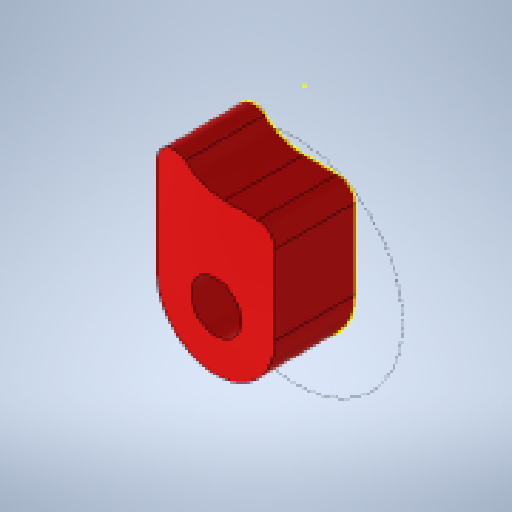
# Autodesk Inventor part: Cam - Lever
Saved by Autodesk Inventor 2023.2 (Build 272271000, 271)
## iProperties
Created: 2024-01-19
Part Number: Cam - Lever
Material: Nylon 6/6
Document SubType Name: Modeling
Designer: Nathan Cai
Density: 1.13 g/cm^3
Appearance: Red
Mass: 0.32887 g
Surface Area: 3.14473 cm^2
Volume: 0.291035 cm^3
Author: Nathan Cai
Autodesk Inventor part; units mm, degrees
ref_plane "YZ Plane" through (0, 0, 0) normal (1, 0, 0) x (0, 1, 0)
ref_plane "XZ Plane" through (0, 0, 0) normal (0, 1, 0) x (-1, 0, 0)
ref_plane "XY Plane" through (0, 0, 0) normal (0, 0, 1) x (1, 0, 0)
sketch "Sketch1" plane through (0, 0, 0) normal (0, 0, 1) x (1, 0, 0)
  circle A0 centre (0, 0) radius 1.5
  circle A1 centre (0, 0) radius 3.5
  circle A2 centre (0, 0) radius 5.75 construction
  line L0 (0, 0) -> (0, 5.75) construction
  circle A3 centre (0.5, 9.2365) radius 3.5
  line L1 (0, 0) -> (0, 5.75) construction
  line L2 (3.5, 0) -> (3.5, 5.75)
  line L3 (-3.5, 5.75) -> (-3.5, 0)
  arc A4 (-3.5, 0) -> (3.5, 0) centre (0, 0) ccw
  arc A5 (3.5, 5.75) -> (-1.9961, 2.875) centre (0, 5.75) ccw
  arc A6 (-3.4062, 0.805) -> (-3.4062, 4.945) centre (-12.1649, 2.875) ccw
  line L4 (0.5, 5.7365) -> (3.5, 5.7365)
  point P0 (0, 2.875)
  point P1 (-3.4345, 6.424)
  point P2 (3.5, 0)
  point P3 (3.244, 7.0639)
  point P4 (-3.5, 0)
  point P5 (-2.744, 7.9226)
  dimension "d2" = 11.5
  dimension "d3" = 7
  dimension "d0" = 3
  dimension "d1" = 7
  dimension "d4" = 3.5
  dimension "d9" = 0.5
  dimension "d10" = 9
  constraints: 12 end point, 11 point on circle, 6 tangent, 5 centre point, 3 coincident, 2 equal length, 1 horizontal, 1 midpoint, 1 perpendicular, 1 point on line, 1 vertical, 1 vertical alignment, 5 other
  measures "d0" diameter of A0
  measures "d1" diameter of A1
  measures "d4" radius of A5
  measures "d9" distance from line of L0 point (0.5, 9.236)
  measures "d10" radius of A6
extrude "Extrusion1" add sketch "Sketch1" along normal blind 4.7625 contours A1 | A1 A5 A3 L4 L2 | A1 A6 A5 | L3 A5 A6 A1
fillet "Fillet1" radius 1 1 edges at (-2.744, 7.9226, 2.3813)
fillet "Fillet2" radius 1 1 edges at (3.5, 5.7365, 2.3813)
sketch "Sketch2" plane through (0, 0, 0) normal (0, 0, -1) x (-1, 0, 0)
  line L0 (-3.5, 0) -> (-3.5, 4.7365) projected
  arc A0 (-3.5, 0) -> (3.5, 0) centre (0, 0) ccw projected
  circle A1 centre (0, 0) radius 1.5 projected
  circle A2 centre (0, 0) radius 6.3558 construction
  arc A3 (3.4953, 5.9311) -> (1.8307, 6.6254) centre (2.4966, 5.8794) ccw projected
  arc A4 (-0.5, 5.7365) -> (1.8307, 6.6254) centre (-0.5, 9.2365) ccw projected
  line L1 (3.5, 5.75) -> (3.5, 0) projected
  line L2 (-2.5, 5.7365) -> (-0.5, 5.7365) projected
  arc A5 (-2.5, 5.7365) -> (-3.5, 4.7365) centre (-2.5, 4.7365) ccw projected
  arc A6 (-2.5, 5.7365) -> (-3.5, 4.7365) centre (-2.5, 4.7365) ccw projected
  arc A7 (3.5, 5.75) -> (3.4953, 5.9311) centre (0, 5.75) ccw projected
  constraints: 1 centre point, 1 coincident, 1 tangent
equation "\"d4\" = 0.5 * d1"
body "Solid1"
